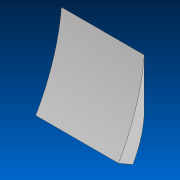
# Autodesk Inventor part: Part1
Saved by Autodesk Inventor 2022 (Build 260153000, 153)
## iProperties
Created: 2022-04-25
Part Number: Part1
Material: Generic
Document SubType Name: Modeling
Designer: score_nygvs6w
Density: 1 g/cm^3
Appearance: Default
Author: score_nygvs6w
Autodesk Inventor part; units mm, degrees
ref_plane "YZ Plane" through (0, 0, 0) normal (1, 0, 0) x (0, 1, 0)
ref_plane "XZ Plane" through (0, 0, 0) normal (0, 1, 0) x (-1, 0, 0)
ref_plane "XY Plane" through (0, 0, 0) normal (0, 0, 1) x (1, 0, 0)
sketch "Sketch1" plane through (0, 0, 0) normal (1, 0, 0) x (0, 1, 0)
  line L0 (-219.6367, 33.4515) -> (-197.6397, 20.7515)
  line L1 (-197.6397, 20.7515) -> (-184.9397, 42.7485)
  line L2 (-184.9397, 42.7485) -> (-206.9367, 55.4485)
  line L3 (-206.9367, 55.4485) -> (-219.6367, 33.4515)
  line L4 (-219.6367, 33.4515) -> (-184.9397, 42.7485) construction
  line L5 (-197.6397, 20.7515) -> (-206.9367, 55.4485) construction
  circle A0 centre (-38.1, 41.275) radius 38.1
  line L6 (0, 0) -> (-228.6, 0)
  line L7 (-228.6, 0) -> (-228.6, -25.4)
  line L8 (-228.6, -25.4) -> (0, -25.4)
  line L9 (0, -25.4) -> (0, 0)
  line L10 (0, 0) -> (-228.6, -25.4) construction
  line L11 (-228.6, 0) -> (0, -25.4) construction
  line L12 (-38.1, 3.175) -> (-132.0434, 3.175)
  arc A1 (-197.6397, 20.7515) -> (-132.0434, 3.175) centre (-132.0434, 134.3676) ccw
  arc A2 (-184.9397, 42.7485) -> (-60.9953, 3.175) centre (-32.1603, 307.3702) ccw
  circle A3 centre (-38.1, 41.275) radius 44.45
  point P0 (-202.2882, 38.1)
  point P1 (-114.3, -12.7)
  dimension "d0" = 76.2
  dimension "d8" = 88.9
  dimension "d1" = 25.4
  dimension "d2" = 60
  dimension "d3" = 41.275
  dimension "d4" = 38.1
  dimension "d5" = 146.847
  dimension "d6" = 20.7515
  dimension "d7" = 228.6
  constraints: 26 end point, 4 midpoint, 4 parallel, 4 point on circle, 3 horizontal, 3 point on line, 3 tangent, 2 centre point, 2 equal length, 2 perpendicular, 1 coincident, 1 vertical alignment, 5 other
  measures "d1" distance of L0.end L1.end
  measures "d2" angle of L1 L6
  measures "d3" distance from line of point (-38.1, 41.275) L6
  measures "d4" distance from line of L9 point (-38.1, 41.275)
  measures "d5" distance of point (-38.1, 41.275) L1.end
  measures "d6" distance from line of L6 L0.end
  measures "d7" distance of L7.end L8.end
extrude "Extrusion1" add sketch "Sketch1" along normal blind 127 contours L1 A2 L12 A1
body "Solid1"
